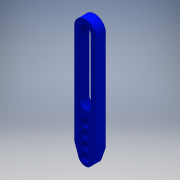
# Autodesk Inventor part: 轉向軸19
Saved by Autodesk Inventor 2019 (Build 230136000, 136)
## iProperties
Created: 2020-03-20
Part Number: 轉向軸19
Material: 一般
Document SubType Name: Modeling
Designer: 吳昇峻
Density: 1 g/cm^3
Appearance: 預設
Author: 吳昇峻
Autodesk Inventor part; units mm, degrees
ref_plane "YZ Plane" through (0, 0, 0) normal (1, 0, 0) x (0, 1, 0)
ref_plane "XZ Plane" through (0, 0, 0) normal (0, 1, 0) x (-1, 0, 0)
ref_plane "XY Plane" through (0, 0, 0) normal (0, 0, 1) x (1, 0, 0)
sketch "草圖1" plane through (0, 0, 0) normal (0, 1, 0) x (-1, 0, 0)
  arc A0 (1.8, 0) -> (-1.8, 0) centre (0, 0) ccw
  line L0 (0, 0) -> (0, -20) construction
  arc A1 (-1.8, -20) -> (1.8, -20) centre (0, -20) ccw
  arc A2 (3.5, 0) -> (-3.5, 0) centre (0, 0) ccw
  line L1 (1.8, 0) -> (1.8, -20)
  line L2 (-1.8, 0) -> (-1.8, -20)
  line L3 (0, -20) -> (0, -35) construction
  line L4 (3.5, 0) -> (3.5, -31.8)
  line L5 (-3.5, 0) -> (-3.5, -31.8)
  circle A3 centre (0, -35) radius 1.25
  line L6 (0, -35) -> (0, -25.4) construction
  line L7 (0, -35) -> (0, -31.8) construction
  line L8 (0, -31.8) -> (0, -28.6) construction
  line L9 (0, -28.6) -> (0, -25.4) construction
  circle A4 centre (0, -31.8) radius 1.25
  circle A5 centre (0, -28.6) radius 1.25
  circle A6 centre (0, -25.4) radius 1.25
  line L10 (3.5, -31.8) -> (2.1243, -35.7414)
  line L11 (-3.5, -31.8) -> (-2.1243, -35.7414)
  arc A7 (-2.1243, -35.7414) -> (2.1243, -35.7414) centre (0, -35) ccw
  dimension "d0" = 3.6
  dimension "d1" = 20
  dimension "d2" = 3.6
  dimension "d3" = 7
  dimension "d5" = 15
  dimension "d9" = 2.5
  dimension "d13" = 3.2
  dimension "d14" = 3.2
  dimension "d15" = 3.2
  dimension "d16" = 2.5
  dimension "d17" = 2.5
  dimension "d18" = 2.5
  constraints: 24 end point, 8 centre point, 8 point on circle, 7 coincident, 4 tangent, 3 point on line, 2 vertical, 1 collinear
  measures "d0" diameter of A0
  measures "d1" distance of L0.start L0.end
  measures "d2" diameter of A1
  measures "d3" diameter of A2
  measures "d5" distance of L3.start L3.end
  measures "d9" diameter of A3
  measures "d13" distance of L6.start L7.end
  measures "d14" distance of L7.end L8.end
  measures "d15" distance of L8.end L6.end
  measures "d16" diameter of A4
  measures "d17" diameter of A5
  measures "d18" diameter of A6
extrude "Extrusion3" add sketch "草圖1" along normal blind 3
body "Solid3"
